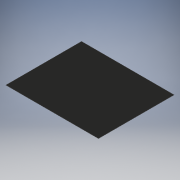
# Autodesk Inventor part: TFT
Saved by Autodesk Inventor 2016 (Build 200138000, 138)
## iProperties
Created: 2016-09-20
Part Number: TFT
Material: 一般
Document SubType Name: Modeling
Designer: KOTA-NPC2
Density: 1 g/cm^3
Appearance: 既定
Author: KOTA-NPC2
Autodesk Inventor part; units mm, degrees
ref_plane "YZ Plane" through (0, 0, 0) normal (1, 0, 0) x (0, 1, 0)
ref_plane "XZ Plane" through (0, 0, 0) normal (0, 1, 0) x (-1, 0, 0)
ref_plane "XY Plane" through (0, 0, 0) normal (0, 0, 1) x (1, 0, 0)
sketch "スケッチ1" plane through (0, 0, 0) normal (0, 0, 1) x (1, 0, 0)
  line L0 (-17.75, 14.5) -> (17.75, 14.5)
  line L1 (17.75, 14.5) -> (17.75, -14.5)
  line L2 (17.75, -14.5) -> (-17.75, -14.5)
  line L3 (-17.75, -14.5) -> (-17.75, 14.5)
  point P0 (0, 0)
  dimension "d14" = 14.5
  dimension "d15" = 14.5
  dimension "d50" = 17.75
  dimension "d51" = 17.75
  constraints: 8 end point, 2 parallel, 1 horizontal, 1 perpendicular
  measures "d14" distance from line of point (0, 0) L0
  measures "d15" distance from line of point (0, 0) L2
  measures "d50" distance from line of point (0, 0) L1
  measures "d51" distance from line of point (0, 0) L3
extrude "押し出し5" add sketch "スケッチ1" along normal blind 0.06
equation "\"d15\" = d14"
equation "\"d51\" = d50"
